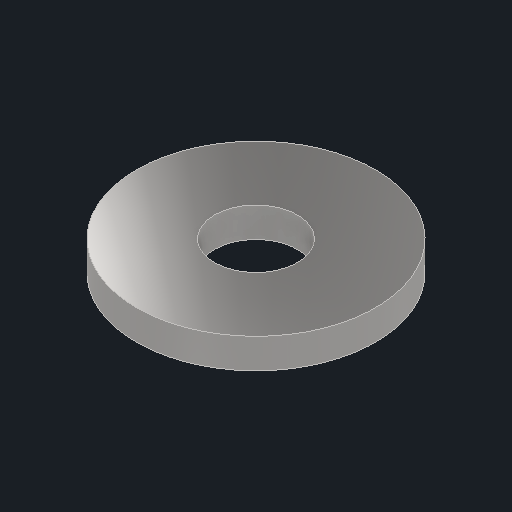
# Autodesk Inventor part: SWasher .500 OD x .062500
Saved by Autodesk Inventor 2025 (Build 290162000, 162)
## iProperties
Created: 2020-06-02
Part Number: SWasher .500 OD x .062500
Material: Steel, Cast
Document SubType Name: Modeling
Designer: yuany
Density: 7.85 g/cm^3
Appearance: Semi-Polished
Author: yuany
Autodesk Inventor part; units mm, degrees
ref_plane "YZ Plane" through (0, 0, 0) normal (1, 0, 0) x (0, 1, 0)
ref_plane "XZ Plane" through (0, 0, 0) normal (0, 1, 0) x (-1, 0, 0)
ref_plane "XY Plane" through (0, 0, 0) normal (0, 0, 1) x (1, 0, 0)
sketch "Sketch1" plane through (0, 0, 0) normal (0, 1, 0) x (-1, 0, 0)
  circle A0 centre (0, 0) radius 2.1971
  circle A1 centre (0, 0) radius 6.35
  dimension "d0" = 4.3942
  dimension "d1" = 12.7
  constraints: 2 centre point, 2 coincident
  measures "d0" diameter of A0
  measures "d1" diameter of A1
extrude "Extrusion1" add sketch "Sketch1" along normal blind 1.5875
body "Solid1"
